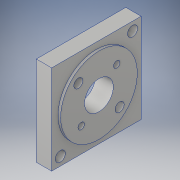
# Autodesk Inventor part: SportMotorBlock
Saved by Autodesk Inventor 2019.4 (Build 234330000, 330)
## iProperties
Created: 2020-02-08
Part Number: SportMotorBlock
Material: Aluminum 6061
Document SubType Name: Modeling
Designer: Paul Lefeuvre
Density: 2.7 g/cm^3
Appearance: Aluminum - Flat
Author: Paul Lefeuvre
Autodesk Inventor part; units mm, degrees
ref_plane "YZ Plane" through (0, 0, 0) normal (1, 0, 0) x (0, 1, 0)
ref_plane "XZ Plane" through (0, 0, 0) normal (0, 1, 0) x (-1, 0, 0)
ref_plane "XY Plane" through (0, 0, 0) normal (0, 0, 1) x (1, 0, 0)
sketch "Sketch1" plane through (0, 0, 0) normal (1, 0, 0) x (0, 1, 0)
  line L0 (-22.225, 22.225) -> (22.225, 22.225)
  line L1 (22.225, 22.225) -> (22.225, -22.225)
  line L2 (22.225, -22.225) -> (-22.225, -22.225)
  line L3 (-22.225, -22.225) -> (-22.225, 22.225)
  line L4 (-22.225, 22.225) -> (22.225, -22.225) construction
  line L5 (22.225, 22.225) -> (-22.225, -22.225) construction
  circle A0 centre (0, 0) radius 19.05
  circle A1 centre (0, 0) radius 7.1374
  circle A2 centre (0, 0) radius 12.4968 construction
  circle A3 centre (0, 0) radius 14.5 construction
  circle A4 centre (8.8366, -8.8366) radius 1.6002
  circle A5 centre (-8.8366, 8.8366) radius 1.6002
  circle A6 centre (10.253, 10.253) radius 2.2479
  circle A7 centre (-10.253, -10.253) radius 2.2479
  circle A8 centre (0, 0) radius 25.4 construction
  circle A9 centre (-17.9605, 17.9605) radius 2.5
  circle A10 centre (17.9605, -17.9605) radius 2.5
  dimension "d0" = 44.45
  dimension "d1" = 44.45
  dimension "d2" = 38.1
  dimension "d4" = 14.2748
  dimension "d5" = 24.9936
  dimension "d6" = 29
  dimension "d7" = 3.2004
  dimension "d8" = 3.2004
  dimension "d9" = 4.4958
  dimension "d10" = 4.4958
  dimension "d11" = 50.8
  dimension "d12" = 5
  dimension "d13" = 5
  constraints: 12 end point, 11 centre point, 6 point on circle, 6 point on line, 5 coincident, 2 midpoint, 2 parallel, 1 horizontal, 1 perpendicular
  measures "d0" distance of L1.end L2.end
  measures "d1" distance of L0.end L1.end
  measures "d2" diameter of A0
  measures "d4" diameter of A1
  measures "d5" diameter of A2
  measures "d6" diameter of A3
  measures "d7" diameter of A4
  measures "d8" diameter of A5
  measures "d9" diameter of A6
  measures "d10" diameter of A7
  measures "d11" diameter of A8
  measures "d12" diameter of A9
  measures "d13" diameter of A10
extrude "Extrusion1" add sketch "Sketch1" along normal blind 7.62 contours L0 L1 L2 L3 | A0
extrude "Extrusion2" add sketch "Sketch1" along normal blind 8.89 contours A0
body "Solid1"
